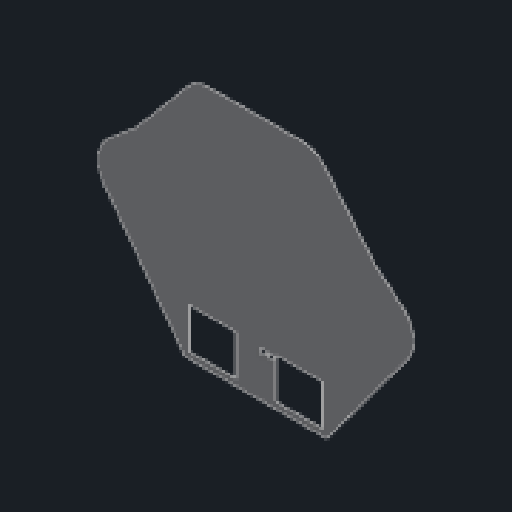
# Autodesk Inventor part: ChestFrontPanel
Saved by Autodesk Inventor 2025.2 (Build 292293000, 293)
## iProperties
Created: 2025-09-23
Part Number: ChestFrontPanel
Material: Generic
Document SubType Name: Sheet Metal
Designer: valer
Density: 1 g/cm^3
Sheet Metal Rule: Default_mm
Appearance: Default
Author: valer
Autodesk Inventor part; units mm, degrees
ref_plane "YZ Plane" through (0, 0, 0) normal (1, 0, 0) x (0, 1, 0)
ref_plane "XZ Plane" through (0, 0, 0) normal (0, 1, 0) x (-1, 0, 0)
ref_plane "XY Plane" through (0, 0, 0) normal (0, 0, 1) x (1, 0, 0)
sketch "Sketch1" plane through (0, 0, 0) normal (0, 0, 1) x (1, 0, 0)
  line L0 (-341.7653, 0) -> (341.7653, 0) construction
  line L1 (0, -75.5138) -> (0, 453.0828) construction
  line L2 (183.676, 264.154) -> (223.6199, 230.6371) construction
  arc A0 (180.154, 267.676) -> (183.676, 264.154) centre (202.0437, 286.0437) ccw construction
  line L3 (105.6111, 356.5128) -> (180.154, 267.676) construction
  arc A1 (105.6111, 356.5128) -> (69.1282, 373.525) centre (69.1282, 325.9) ccw construction
  line L4 (-69.1282, 373.525) -> (69.1282, 373.525) construction
  arc A2 (231.2425, 165.7605) -> (223.6199, 230.6371) centre (193.0071, 194.1542) ccw construction
  line L5 (231.2425, 165.7605) -> (183.8243, 101.9065) construction
  line L6 (0, 373.525) -> (69.1282, 373.525) construction
  line L7 (183.8243, 101.9065) -> (108.1482, 0) construction
  line L8 (108.1482, 0) -> (0, 0) construction
  line L9 (-183.676, 264.154) -> (-223.6199, 230.6371) construction
  arc A3 (-183.676, 264.154) -> (-180.154, 267.676) centre (-202.0437, 286.0437) ccw construction
  line L10 (-105.6111, 356.5128) -> (-180.154, 267.676) construction
  arc A4 (-69.1282, 373.525) -> (-105.6111, 356.5128) centre (-69.1282, 325.9) ccw construction
  arc A5 (-223.6199, 230.6371) -> (-231.2425, 165.7605) centre (-193.0071, 194.1542) ccw construction
  line L11 (-231.2425, 165.7605) -> (-183.8243, 101.9065) construction
  line L12 (0, 373.525) -> (-69.1282, 373.525) construction
  line L13 (-183.8243, 101.9065) -> (-108.1482, 0) construction
  line L14 (-108.1482, 0) -> (0, 0) construction
  circle A6 centre (20.5, 100) radius 3
  line L15 (20.5, 100) -> (8, 100) construction
  line L16 (8, 100) -> (0, 100) construction
  circle A7 centre (8, 100) radius 3
  circle A8 centre (-20.5, 100) radius 3
  line L17 (-20.5, 100) -> (-8, 100) construction
  circle A9 centre (-8, 100) radius 3
  circle A10 centre (90, 16) radius 1.5
  circle A11 centre (90, 65) radius 1.5
  circle A12 centre (41, 16) radius 1.5
  circle A13 centre (41, 65) radius 1.5
  circle A14 centre (65.5, 40.5) radius 25.5 construction
  arc A15 (101, 69) -> (99, 71) centre (99, 69) ccw construction
  line L18 (32, 71) -> (99, 71) construction
  arc A16 (32, 71) -> (30, 69) centre (32, 69) ccw construction
  line L19 (30, 12) -> (30, 69) construction
  arc A17 (30, 12) -> (32, 10) centre (32, 12) ccw construction
  line L20 (99, 10) -> (32, 10) construction
  arc A18 (99, 10) -> (101, 12) centre (99, 12) ccw construction
  line L21 (101, 69) -> (101, 12) construction
  circle A19 centre (-41, 16.5) radius 1.5
  circle A20 centre (-41, 65.5) radius 1.5
  circle A21 centre (-90, 16.5) radius 1.5
  circle A22 centre (-90, 65.5) radius 1.5
  circle A23 centre (-65.5, 41) radius 25.5 construction
  arc A24 (-30, 69.5) -> (-32, 71.5) centre (-32, 69.5) ccw construction
  line L22 (-99, 71.5) -> (-32, 71.5) construction
  arc A25 (-99, 71.5) -> (-101, 69.5) centre (-99, 69.5) ccw construction
  line L23 (-101, 12.5) -> (-101, 69.5) construction
  arc A26 (-101, 12.5) -> (-99, 10.5) centre (-99, 12.5) ccw construction
  line L24 (-32, 10.5) -> (-99, 10.5) construction
  arc A27 (-32, 10.5) -> (-30, 12.5) centre (-32, 12.5) ccw construction
  line L25 (-30, 69.5) -> (-30, 12.5) construction
  line L26 (108.1482, 0) -> (-108.1482, 0)
  line L27 (-108.1482, 0) -> (-193.5475, 115)
  line L28 (-193.5475, 115) -> (193.5475, 115)
  line L29 (193.5475, 115) -> (108.1482, 0)
  circle A28 centre (-65.5, 41) radius 26.5
  circle A29 centre (65.5, 40.5) radius 26.5
  point P0 (0, 0)
  point P1 (0, 115)
  dimension "d6" = 6
  dimension "d7" = 8
  dimension "d8" = 12.5
  dimension "d9" = 100
  dimension "d10" = 15
  dimension "d15" = 1
  dimension "d16" = 1
  measures "d6" diameter of A6
  measures "d7" distance of L15.end L16.end
  measures "d8" distance of L15.start L15.end
  measures "d9" distance between parallel lines of L8 L15
  measures "d10" distance between parallel lines of L28 L15
  measures "d15" radial gap between concentric circles of A28 A23
  measures "d16" radial gap between concentric circles of A29 A14
extrude "Plate1" add sketch "Sketch1" along normal blind 2.54
chamfer "Chamfer1" distance 40 angle 45 2 edges at (-193.5475, 115, 1.27) (193.5475, 115, 1.27)
fillet "Fillet1" radius 4 4 edges at (108.1482, 0, 1.27) (169.6998, 82.8863, 1.27) (-108.1482, 0, 1.27) (-169.6998, 82.8863, 1.27)
sketch "Sketch2" plane through (0, 0, 0) normal (0, 0, -1) x (-1, 0, 0)
  line L0 (-153.5475, 115) -> (153.5475, 115)
  line L1 (-153.5475, 115) -> (-89.2554, 369.0629)
  line L2 (0, -52.9429) -> (0, 317.6573) construction
  line L3 (-89.2554, 369.0629) -> (0, 369.0629)
  arc A0 (-69.1282, 373.525) -> (-105.6111, 356.5128) centre (-69.1282, 325.9) ccw construction
  line L4 (153.5475, 115) -> (89.2554, 369.0629)
  line L5 (89.2554, 369.0629) -> (0, 369.0629)
  point P0 (0, 0)
sheet face with bend "Face2" sketch "Sketch2" thickness 2.54 toward (0, 0, 1) bend radius 2.54 relief straight relief width 2.54 relief depth 1.27
bend "Bend1"
fillet "Fillet2" radius 16 2 edges at (89.2554, 369.0629, 1.27) (-89.2554, 369.0629, 1.27)
equation "\"d0\" = Thickness"
equation "\"d17\" = BendRadius"
equation "\"d18\" = BendReliefWidth"
equation "\"d20\" = MinimumRemnant"
equation "\"d19\" = BendReliefDepth"
equation "\"d21\" = TransitionRadius"
equation "\"BendRadius\" = Thickness"
equation "\"BendReliefWidth\" = Thickness"
equation "\"BendReliefDepth\" = 0.5 * Thickness"
equation "\"CornerReliefSize\" = 4 * Thickness"
equation "\"MinimumRemnant\" = 2 * Thickness"
equation "\"TransitionRadius\" = BendRadius"
equation "\"JacobiRadiusSize\" = BendRadius"
equation "\"GapSize\" = Thickness"
equation "\"Thickness\" = 2.54"
body "Solid1"
